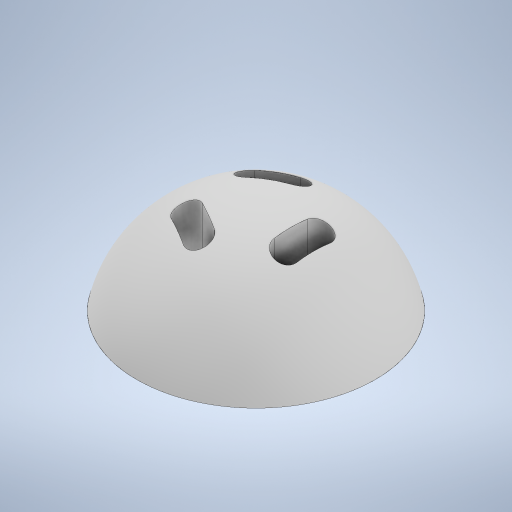
# Autodesk Inventor part: hemisphere_2
Saved by Autodesk Inventor 2024.2 (Build 282272000, 272)
## iProperties
Created: 2024-06-17
Part Number: hemisphere_2
Material: Ogólny
Document SubType Name: Modeling
Designer: Konrad
Density: 1 g/cm^3
Appearance: Domyślna
Author: Konrad
Autodesk Inventor part; units mm, degrees
ref_plane "YZ Plane" through (0, 0, 0) normal (1, 0, 0) x (0, 1, 0)
ref_plane "XZ Plane" through (0, 0, 0) normal (0, 1, 0) x (-1, 0, 0)
ref_plane "XY Plane" through (0, 0, 0) normal (0, 0, 1) x (1, 0, 0)
sketch "Szkic1" plane through (0, 0, 0) normal (0, 1, 0) x (-1, 0, 0)
  circle A0 centre (0, 0) radius 14.1 construction
  line L0 (0, 0) -> (-14.1, 0) construction
  circle A1 centre (0, 0) radius 22.5 construction
  circle A2 centre (-13.2497, 4.8225) radius 1.75
  circle A3 centre (-13.2497, -4.8225) radius 1.75
  circle A4 centre (2.4484, 13.8858) radius 1.75
  circle A5 centre (10.8012, 9.0633) radius 1.75
  circle A6 centre (10.8012, -9.0633) radius 1.75
  circle A7 centre (2.4484, -13.8858) radius 1.75
  circle A8 centre (0, 0) radius 35
  circle A9 centre (-13.2497, 4.8225) radius 3.25
  circle A10 centre (-13.2497, -4.8225) radius 3.25
  circle A11 centre (2.4484, -13.8858) radius 3.25
  circle A12 centre (10.8012, -9.0633) radius 3.25
  circle A13 centre (10.8012, 9.0633) radius 3.25
  circle A14 centre (2.4484, 13.8858) radius 3.25
  line L1 (-9.9997, -4.8225) -> (-9.9997, 4.8225)
  line L2 (-16.4997, 4.8225) -> (-16.4997, -4.8225)
  line L3 (4.0734, -16.7004) -> (12.4262, -11.8779)
  line L4 (9.1762, -6.2487) -> (0.8234, -11.0712)
  line L5 (12.4262, 11.8779) -> (4.0734, 16.7004)
  line L6 (0.8234, 11.0712) -> (9.1762, 6.2487)
  dimension "d0" = 28.2
  dimension "d1" = 3.5
  dimension "d2" = 40
  dimension "d5" = 360
  dimension "d7" = 45
  dimension "d8" = 70
  dimension "d12" = 6.5
  dimension "d15" = 360
  dimension "d29" = 360
  constraints: 15 centre point, 14 end point, 7 point on circle, 5 coincident, 4 tangent, 2 equal radius, 1 horizontal, 1 symmetric about line, 45 other
  measures "d0" diameter of A0
  measures "d1" diameter of A2
  measures "d7" diameter of A1
  measures "d8" diameter of A8
  measures "d12" diameter of A9
sketch "Szkic3" plane through (0, 0, 0) normal (0, 0, 1) x (1, 0, 0)
  arc A0 (0, 35) -> (-35, 0) centre (0, 0) ccw
  line L0 (0, 35) -> (0, 0)
  line L1 (0, 0) -> (-35, 0)
  line L2 (0, -8.4497) -> (0, 50.6985) projected
  dimension "d19" = 35
  constraints: 4 end point, 2 point on circle, 1 centre point, 1 coincident, 1 perpendicular, 1 vertical
  measures "d19" radius of A0
revolve "Obrót1" add sketch "Szkic3" angle 360 about axis through (0, -10, 0) along (0, 1, 0)
extrude "Wyciągnięcie proste1" cut sketch "Szkic1" along normal through all contours A2 | A3 | A4 | A5 | A6 | A7 | A9 | L1 A10 L2 A9 | A10 | A11 | A11 L4 A12 L3 | A12 | A13 | A13 L6 A14 L5 | A14
extrude "Wyciągnięcie proste2" add sketch "Szkic1" along normal blind 17.85 contours A9 | L1 A10 L2 A9 | A10 | A11 | A11 L4 A12 L3 | A12 | A13 | A13 L6 A14 L5 | A14
extrude "Wyciągnięcie proste3" cut sketch "Szkic1" along normal blind 7.85 contours A2 | A3 | A4 | A5 | A6 | A7 | A8 | A9 | L1 A10 L2 A9 | A10 | A11 | A11 L4 A12 L3 | A12 | A13 | A13 L6 A14 L5 | A14
